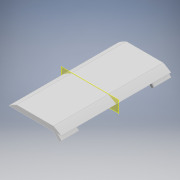
# Autodesk Inventor part: Case_Side_Screw
Saved by Autodesk Inventor 2020 (Build 240168000, 168)
## iProperties
Created: 2020-07-28
Part Number: Case_Side_Screw
Material: 일반
Document SubType Name: Modeling
Designer: Knowblesse
Density: 1 g/cm^3
Appearance: 기본값
Author: Knowblesse
## iProperties of the stored document _3D 인쇄.ipt
Created: 2020-07-28
Part Number: _3D 인쇄
Material: 일반
Document SubType Name: Modeling
Designer: Knowblesse
Density: 1 g/cm^3
Appearance: 기본값
Author: Knowblesse
Autodesk Inventor part; units mm, degrees
ref_plane "YZ Plane" through (0, 0, 0) normal (1, 0, 0) x (0, 1, 0)
ref_plane "XZ Plane" through (0, 0, 0) normal (0, 1, 0) x (-1, 0, 0)
ref_plane "XY Plane" through (0, 0, 0) normal (0, 0, 1) x (1, 0, 0)
sketch "스케치1" plane through (0, 0, 0) normal (0, 0, 1) x (1, 0, 0)
  arc A0 (4.665, 5.9998) -> (-4.665, 5.9998) centre (0, 0) ccw
  line L0 (4.665, 5.9998) -> (-4.665, 5.9998)
  line L1 (-3.3945, 6.7998) -> (3.3945, 6.7998)
  arc A1 (4.5335, 5.9998) -> (-4.5335, 5.9998) centre (0, -0.1) ccw
  point P0 (0, 7.6)
  point P1 (3.1863, 6.7998)
  point P2 (-3.1863, 6.7998)
  dimension "d1" = 7.6
  dimension "d2" = 9.33
  dimension "d5" = 0.8
  dimension "d6" = 7.6
  dimension "d7" = 0.1
  constraints: 7 point on circle, 4 end point, 2 centre point, 2 point on line, 2 vertical alignment, 1 coincident, 1 parallel
  measures "d1" radius of A0
  measures "d2" distance of L0.start L0.end
  measures "d5" distance between parallel lines of L0 L1
  measures "d6" radius of A1
  measures "d7" distance of point (0, 0) A1.centre
extrude "돌출1" add sketch "스케치1" along normal blind 19 contours L0 A1 L1
sketch "스케치2" plane through (0, 0, 19) normal (0, 0, 1) x (1, 0, 0)
  line L0 (-4.5335, 5.9998) -> (4.5335, 5.9998) projected
  line L1 (3.8635, 5.9998) -> (4.5706, 5.2927)
  line L2 (4.5706, 5.2927) -> (4.217, 4.9392)
  line L3 (4.217, 4.9392) -> (3.1564, 5.9998)
  point P0 (0, 0)
  dimension "d8" = 0.67
  dimension "d9" = 45
  dimension "d10" = 0.5
  dimension "d11" = 1
  constraints: 6 end point, 2 point on line, 1 parallel, 1 perpendicular
  measures "d8" distance of L1.start L0.end
  measures "d9" angle of L0 L1
  measures "d10" distance of L1.end L2.end
  measures "d11" distance from line of L1.start L2
extrude "돌출2" add sketch "스케치2" against normal blind 3
ref_plane "작업 평면1" through (0, 0, 9.5) normal (0, 0, 1) x (1, 0, 0)
mirror "미러1" about plane through (0, 0, 9.5) normal (0, 0, 1) of "돌출2"
